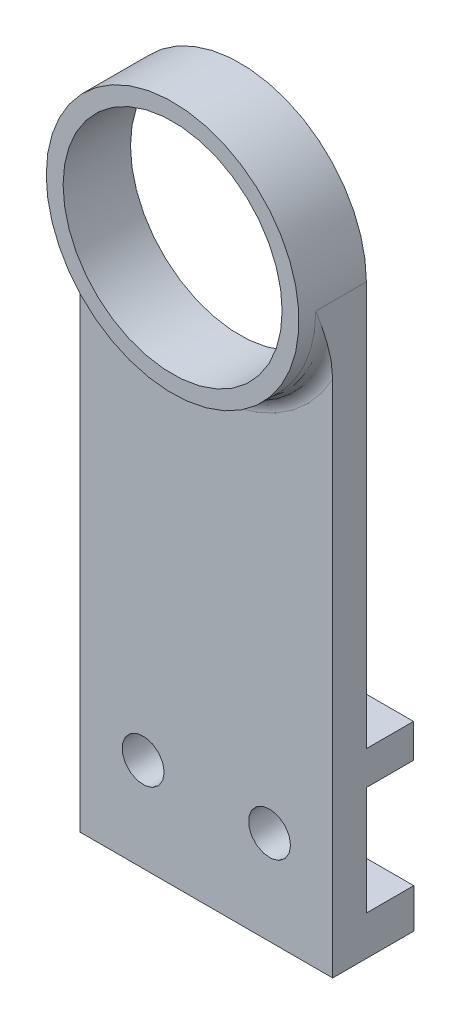
# Autodesk Inventor part: Layer2RodHolder
Saved by Autodesk Inventor 2025 (Build 290162000, 162)
## iProperties
Created: 2025-01-12
Part Number: Layer2RodHolder
Material: Generic
Document SubType Name: Modeling
Designer: Trevor
Density: 1 g/cm^3
Appearance: Default
Author: Trevor
Autodesk Inventor part; units mm, degrees
ref_plane "YZ Plane" through (0, 0, 0) normal (1, 0, 0) x (0, 1, 0)
ref_plane "XZ Plane" through (0, 0, 0) normal (0, 1, 0) x (-1, 0, 0)
sketch "Sketch1" plane through (0, 0, 0) normal (0, 0, 1) x (1, 0, 0)
  circle A0 centre (9.3084, 52.0833) radius 13 projected
  line L0 (-18, -12.7) -> (-18, 0) projected
  line L1 (76.6, -12.7) -> (-18, -12.7) projected
  line L2 (76.6, 0) -> (76.6, -12.7) projected
  line L3 (-18, 0) -> (76.6, 0) projected
  circle A1 centre (9.3084, 52.0833) radius 15
  line L4 (9.3084, 52.0833) -> (-5.6916, 52.0833) construction
  line L5 (9.3084, 52.0833) -> (24.3084, 52.0833) construction
  line L6 (24.3084, 52.0833) -> (24.3084, 0)
  line L7 (-5.6916, 52.0833) -> (-5.6916, 0)
  point P0 (0, 0)
  dimension "d0" = 2
  constraints: 8 end point, 3 point on line, 2 perpendicular, 2 point on circle, 1 centre point, 1 tangent
  measures "d0" radial gap between concentric circles of A0 A1
ref_plane "Work Plane1" through (0, 0, 0) normal (0, 0, 1) x (1, 0, 0)
sketch "Sketch2" plane through (0, 0, 0) normal (0, 0, 1) x (1, 0, 0)
  point P0 (0, 0)
extrude "Extrusion1" add sketch "Sketch1" along normal blind 4 contours L7 A1 L6 L3 | A1
sketch "Sketch3" plane through (24.3084, 0, 0) normal (1, 0, 0) x (0, 0, -1)
  line L0 (5.625, -50.2216) -> (5.625, -17.4784) projected
  line L1 (0, 0) -> (-4, 0) projected
  line L2 (-4, 0) -> (-4, -17.4784)
  line L3 (-4, -17.4784) -> (5.625, -17.4784)
  line L4 (5, -12.7) -> (0, -12.7) projected
  line L5 (5, -12.7) -> (42.625, -12.7) projected
  line L6 (5.625, -17.4784) -> (5.625, -12.8)
  line L7 (5.625, -12.8) -> (0, -12.8)
  line L8 (0, 0) -> (0, -12.7)
  line L9 (5, 0) -> (42.625, 0) projected
  line L10 (5.5947, 0.1) -> (-0.3708, 0.1)
  line L11 (-0.3708, 0.1) -> (-0.3708, 4.1)
  line L12 (-0.3708, 4.1) -> (5.5947, 4.1)
  line L13 (5.5947, 4.1) -> (5.5947, 0.1)
  line L14 (0, 4.1) -> (0, 0)
  line L15 (0, 0) -> (0, -12.7) projected
  line L16 (0, -12.8) -> (0, -12.7)
  point P0 (5.625, -13.7893)
  point P1 (0, 0.1)
  dimension "d3" = 0.1
  dimension "d4" = 0.1
  dimension "d5" = 4
  constraints: 22 end point, 4 perpendicular, 4 vertical, 2 parallel, 1 horizontal, 1 point on line, 1 other
  measures "d3" distance from line of L5 L6.end
  measures "d4" distance from line of L9 L10.start
  measures "d5" distance of L10.end L11.end
extrude "Extrusion2" add sketch "Sketch3" against normal up to surface (30 mm away) contours L8 L16 L7 L6 L3 L2 L1 | L10 L14 L12 L13
sketch "Sketch4" plane through (0, 0, 4) normal (0, 0, 1) x (1, 0, 0)
  point P0 (0, 0)
sketch "Sketch5" plane through (0, 0, 4) normal (0, 0, 1) x (1, 0, 0)
  line L0 (24.3084, 52.0833) -> (24.3084, -17.4784) projected
  arc A0 (24.3084, 52.0833) -> (-5.6916, 52.0833) centre (9.3084, 52.0833) ccw projected
  line L1 (-5.6916, 52.0833) -> (-5.6916, -17.4784) projected
  line L2 (24.3084, -17.4784) -> (-5.6916, -17.4784) projected
  circle A1 centre (9.3084, 52.0833) radius 13 projected
  circle A2 centre (9.3084, 52.0833) radius 15
  point P0 (0, 0)
  point P1 (-5.6916, 52.0833)
  constraints: 1 centre point, 1 coincident
ref_plane "Work Plane2" through (-7.7853, 34.9896, 8) normal (0, 0, 1) x (0.9177573, -0.3971417, 0)
extrude "Extrusion3" add sketch "Sketch5" along normal up to surface (4 mm away) contours A2 A0
fillet "Fillet1" radius 2 1 edges at (9.3084, 37.0833, 4)
sketch "Sketch6" plane through (0, 0, 4) normal (0, 0, 1) x (1, 0, 0)
  line L0 (-5.6916, 0.1) -> (24.3084, 0.1) projected
  line L1 (9.3084, 0.1) -> (9.3084, -12.8) construction
  line L2 (24.3084, -12.8) -> (-5.6916, -12.8) projected
  line L3 (-5.6916, 0.1) -> (-5.6916, -12.8) projected
  line L4 (-5.6916, -6.35) -> (9.3084, -6.35)
  line L5 (-5.6916, -6.35) -> (1.8084, -6.35)
  circle A0 centre (1.8084, -6.35) radius 2.5
  circle A1 centre (16.8084, -6.35) radius 2.5
  point P0 (0, 0)
  dimension "d11" = 5
  constraints: 6 end point, 5 midpoint, 2 centre point, 1 coincident, 1 symmetric about line, 1 other
  measures "d11" diameter of A0
extrude "Extrusion4" cut sketch "Sketch6" against normal blind 10
body "Solid1"
